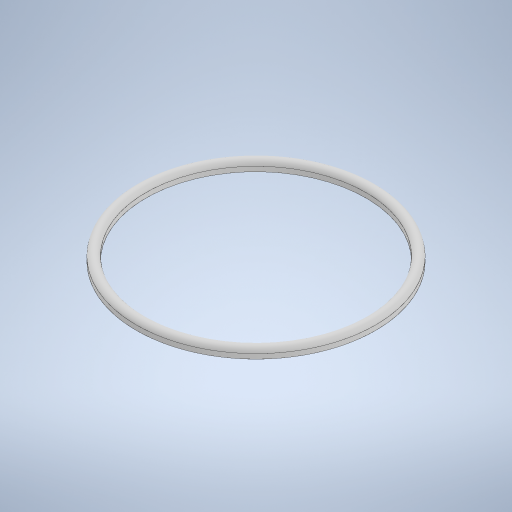
# Autodesk Inventor part: o-ring
Saved by Autodesk Inventor 2023 (Build 270158030, 158C)
## iProperties
Created: 2022-10-27
Part Number: o-ring
Material: Generic
Document SubType Name: Modeling
Designer: cjj5381
Density: 1 g/cm^3
Appearance: Default
Author: cjj5381
Autodesk Inventor part; units mm, degrees
ref_plane "YZ Plane" through (0, 0, 0) normal (1, 0, 0) x (0, 1, 0)
ref_plane "XZ Plane" through (0, 0, 0) normal (0, 1, 0) x (-1, 0, 0)
ref_plane "XY Plane" through (0, 0, 0) normal (0, 0, 1) x (1, 0, 0)
sketch "Sketch1" plane through (0, 0, 0) normal (0, 0, 1) x (1, 0, 0)
  line L0 (0, 0) -> (0, 19.685)
  line L1 (36.5125, 0) -> (39.6875, 0)
  line L2 (39.6875, 0) -> (39.6875, 1.5875)
  line L3 (36.5125, 1.5875) -> (36.5125, 0)
  arc A0 (39.6875, 1.5875) -> (36.5125, 1.5875) centre (38.1, 1.5875) ccw
  point P0 (38.1, 3.175)
  dimension "d0" = 3.175
  dimension "d1" = 76.2
  dimension "d3" = 3.175
  constraints: 8 end point, 3 point on circle, 2 tangent, 1 centre point, 1 horizontal, 1 horizontal alignment, 1 parallel, 1 perpendicular, 1 vertical
  measures "d0" distance from line of L1 point (38.1, 3.175)
  measures "d1" diameter of A0.centre L0
  measures "d3" distance of L1.start L1.end
revolve "Revolution1" add sketch "Sketch1" angle 360 about axis through (0, 0, 0) along (0, 1, 0)
body "Solid1"
